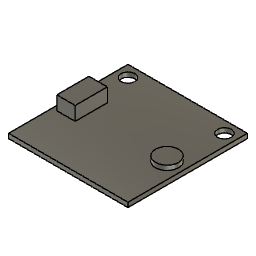
senseEle_PCB_Antenna_rev1_Enclosure_V3 (Autodesk Fusion 360 archive; units mm, degrees)
design "Untitled"
Autodesk Fusion 360 part; units mm, degrees
sketch "Sketch1" plane through (0, 0, 0) normal (0, 0, 1) x (1, 0, 0)
  line L0 (0, 0) -> (26, 0)
  line L1 (26, 0) -> (26, 26)
  line L2 (26, 26) -> (0, 26)
  line L3 (0, 26) -> (0, 0)
  dimension "d1" = 26
  dimension "d2" = 26
  constraint horizontal L0
  constraint vertical L1
  constraint horizontal L2
  constraint vertical L3
  constraint coincident L0.start L3.end
  measures "d1" distance of L0.start L2.end
  measures "d2" distance of L0.start L0.end
  measures "d7" distance of L0.start
extrude "Extrude1" add sketch "Sketch1" along normal blind 1
sketch "Sketch2" plane through (0, 0, 1) normal (0, 0, 1) x (-1, 0, 0)
  line L0 (0, -26) -> (0, 0)
  line L1 (0, 0) -> (-26, 0)
  line L2 (-26, 0) -> (-26, -26)
  line L3 (-26, -26) -> (0, -26)
  circle A0 centre (-23.5, -23.5) radius 1.5
  circle A1 centre (-2.5, -23.5) radius 1.5
  dimension "d5" = 3
  dimension "d6" = 3
  dimension "d7" = 2.5
  dimension "d8" = 2.5
  dimension "d9" = 2.5
  dimension "d10" = 2.5
  measures "d5" diameter of A0
  measures "d6" diameter of A1
  measures "d7" distance of L2 A0.centre
  measures "d8" distance of L0 A1.centre
  measures "d9" distance of L3 A1.centre
  measures "d10" distance of L3 A0.centre
extrude "Extrude2" cut sketch "Sketch2" against normal blind 4 contours A0 | A1
sketch "Sketch3" plane through (0, 0, 1) normal (0, 0, 1) x (-1, 0, 0)
  circle A0 centre (-2.5, -23.5) radius 1.5
  circle A1 centre (-23.5, -23.5) radius 1.5
  line L0 (0, -26) -> (0, 0)
  line L1 (0, 0) -> (-26, 0)
  line L2 (-26, 0) -> (-26, -26)
  line L3 (-26, -26) -> (0, -26)
  line L4 (-1, -16.5) -> (-5, -16.5)
  line L5 (-5, -16.5) -> (-5, -9.5)
  line L6 (-5, -9.5) -> (-1, -9.5)
  line L7 (-1, -9.5) -> (-1, -16.5)
  dimension "d13" = 7
  dimension "d14" = 4
  dimension "d15" = 1
  constraint horizontal L4
  constraint vertical L5
  constraint horizontal L6
  constraint vertical L7
  measures "d13" distance of L4.start L6.end
  measures "d14" distance of L4.start L4.end
  measures "d15" distance of L0 L7
extrude "Extrude3" add sketch "Sketch3" along normal blind 3 contours L4 L5 L6 L7
sketch "Sketch4" plane through (0, 0, 1) normal (0, 0, 1) x (-1, 0, 0)
  line L0 (-1, -9.5) -> (-1, -16.5)
  line L1 (-1, -16.5) -> (-5, -16.5)
  line L2 (-5, -16.5) -> (-5, -9.5)
  line L3 (-5, -9.5) -> (-1, -9.5)
  circle A0 centre (-2.5, -23.5) radius 1.5
  circle A1 centre (-23.5, -23.5) radius 1.5
  line L4 (0, -26) -> (0, 0)
  line L5 (0, 0) -> (-26, 0)
  line L6 (-26, 0) -> (-26, -26)
  line L7 (-26, -26) -> (0, -26)
  circle A2 centre (-22.5, -12) radius 2.5
  dimension "d19" = 5
  dimension "d20" = 3.5
  measures "d19" diameter of A2
  measures "d20" distance of L6 A2.centre
extrude "Extrude4" add sketch "Sketch4" along normal blind 1 contours A2
